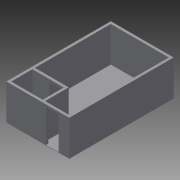
# Autodesk Inventor part: 289 Manning Basement
Saved by Autodesk Inventor 2013 SP2 (Build 170200200, 200)
## iProperties
Created: 2014-06-09
Part Number: 289 Manning Basement
Material: Generic
Document SubType Name: Modeling
Designer: jmw3
Density: 1 g/cm^3
Author: jmw3
Autodesk Inventor part; units mm, degrees
ref_plane "YZ Plane" through (0, 0, 0) normal (1, 0, 0) x (0, 1, 0)
ref_plane "XZ Plane" through (0, 0, 0) normal (0, 1, 0) x (-1, 0, 0)
ref_plane "XY Plane" through (0, 0, 0) normal (0, 0, 1) x (1, 0, 0)
sketch "Sketch1" plane through (0, 0, 0) normal (0, 1, 0) x (-1, 0, 0)
  line L0 (1955.8, -3251.2) -> (-1955.8, -3251.2)
  line L1 (-1955.8, -3251.2) -> (-1955.8, 3251.2)
  line L2 (1955.8, 3251.2) -> (1955.8, -3251.2)
  line L3 (2738.12, 0) -> (-2738.12, 0) projected
  line L4 (0, -4551.68) -> (0, 4551.68) projected
  line L5 (1803.4, -3098.8) -> (-1803.4, -3098.8)
  line L6 (-1803.4, -3098.8) -> (-1803.4, 3098.8)
  line L7 (-152.4, 3098.8) -> (-152.4, 1778)
  line L8 (-304.8, 1625.6) -> (-304.8, 3098.8)
  line L9 (-508, 3098.8) -> (-508, 3251.2)
  line L10 (-1295.4, 3098.8) -> (-1295.4, 3251.2)
  line L11 (-1803.4, 3098.8) -> (-1295.4, 3098.8)
  line L12 (-1955.8, 3251.2) -> (-1295.4, 3251.2)
  line L13 (-508, 3251.2) -> (1955.8, 3251.2)
  line L14 (-508, 3098.8) -> (-304.8, 3098.8)
  line L15 (-152.4, 3098.8) -> (1803.4, 3098.8)
  line L16 (762, 1625.6) -> (762, 1778)
  line L17 (0, 1625.6) -> (0, 1778)
  line L18 (1803.4, 1625.6) -> (762, 1625.6)
  line L19 (0, 1625.6) -> (-304.8, 1625.6)
  line L20 (-152.4, 1778) -> (0, 1778)
  line L21 (762, 1778) -> (1803.4, 1778)
  line L22 (1803.4, 3098.8) -> (1803.4, 1778)
  line L23 (1803.4, 1625.6) -> (1803.4, -3098.8)
  point P0 (0, 0)
  dimension "d0" = 3911.6
  dimension "d3" = 152.4
  dimension "d4" = 152.4
  dimension "d6" = 152.4
  dimension "d11" = 508
  dimension "d12" = 787.4
  dimension "d14" = 6502.4
  dimension "d16" = 152.4
  dimension "d17" = 152.4
  dimension "d19" = 1473.2
  dimension "d20" = 152.4
  dimension "d21" = 762
  dimension "d22" = 1498.6
  dimension "d25" = 1193.8
  constraints: 44 end point, 17 perpendicular, 10 parallel, 5 collinear, 2 horizontal, 3 other
  measures "d0" distance between parallel lines of L2 L1
  measures "d3" distance between parallel lines of L1 L6
  measures "d4" distance between parallel lines of L0 L5
  measures "d6" distance between parallel lines of L8 L7
  measures "d11" distance from line of L6 L10.end
  measures "d12" distance between parallel lines of L9 L10
  measures "d14" distance between parallel lines of L0 L13
  measures "d16" distance between parallel lines of L12 L11
  measures "d17" distance between parallel lines of L18 L21
  measures "d19" distance between parallel lines of L14 L19
  measures "d20" distance between parallel lines of L19 L20
  measures "d21" distance between parallel lines of L17 L16
  measures "d22" distance between parallel lines of L6 L8
  measures "d25" distance between parallel lines of L2 L16
extrude "Extrusion1" add sketch "Sketch1" along normal blind 2184.4 contours L0 L4 L5 L23 L3 L2 | L0 L1 L3 L6 L5 L4 | L3 L23 L18 L16 L21 L22 L15 L4 L13 L2 | L1 L12 L10 L11 L6 L3 | L4 L15 L7 L20 L19 L8 L14 L9 L13
sketch "Sketch2" plane through (0, 0, 0) normal (0, -1, 0) x (1, 0, 0)
  line L0 (-1955.8, 3251.2) -> (1955.8, 3251.2)
  line L1 (1955.8, 3251.2) -> (1955.8, -3251.2)
  line L2 (1955.8, -3251.2) -> (-1955.8, -3251.2)
  line L3 (-1955.8, -3251.2) -> (-1955.8, 3251.2)
  point P0 (0, 0)
  constraints: 8 end point, 2 parallel, 1 horizontal, 1 perpendicular
extrude "Extrusion2" add sketch "Sketch2" along normal blind 25.4
sketch "Sketch3" plane through (0, 2184.4, 0) normal (0, 1, 0) x (1, 0, 0)
  line L0 (-762, -1625.6) -> (0, -1625.6)
  line L1 (0, -1625.6) -> (0, -1778)
  line L2 (0, -1778) -> (-762, -1778)
  line L3 (-762, -1778) -> (-762, -1625.6)
  line L4 (508, -3098.8) -> (1295.4, -3098.8)
  line L5 (1295.4, -3098.8) -> (1295.4, -3251.2)
  line L6 (1295.4, -3251.2) -> (508, -3251.2)
  line L7 (508, -3251.2) -> (508, -3098.8)
  point P0 (0, 0)
  constraints: 16 end point, 4 parallel, 2 horizontal, 2 perpendicular
extrude "Extrusion3" add sketch "Sketch3" against normal blind 152.4
body "Solid1"
